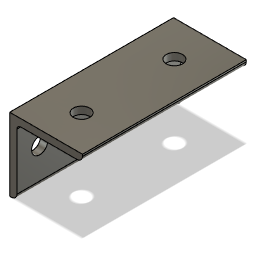
Equerre 80x80x8 longueur 180mm (Autodesk Fusion 360 design; units mm, degrees)
Autodesk Fusion 360 part; units mm, degrees
sketch "Sketch1" plane through (0, 0, 0) normal (0, 0, 1) x (1, 0, 0)
  line L0 (0, 0) -> (0, 80)
  line L1 (0, 80) -> (80, 80)
  line L2 (8, 6) -> (8, 68)
  line L3 (12, 72) -> (74, 72)
  line L4 (80, 78) -> (80, 80)
  line L5 (0, 0) -> (2, 0)
  arc A0 (74, 72) -> (80, 78) centre (74, 78) ccw
  arc A1 (2, 0) -> (8, 6) centre (2, 6) ccw
  arc A2 (12, 72) -> (8, 68) centre (12, 68) ccw
  dimension "d1" = 80
  dimension "d2" = 80
  dimension "d4" = 6
  dimension "d5" = 6
  dimension "d6" = 4
  constraint coincident L0.start L5.start
  constraint horizontal L1
  constraint vertical L0
  constraint perpendicular L1 L4
  constraint perpendicular L2 L5
  constraint parallel L0 L2
  constraint parallel L1 L3
  constraint tangent L3 A0
  constraint tangent L4 A0
  constraint tangent L2 A1
  constraint tangent L5 A1
  constraint tangent L2 A2
  constraint tangent L3 A2
  measures "d1" distance of L0.start L0.end
  measures "d2" distance of L0.end L1.end
  measures "d4" radius of A0
  measures "d5" radius of A1
  measures "d6" radius of A2
extrude "Extrude1" add sketch "Sketch1" along normal mid plane 180
sketch "Sketch2" plane through (0, 0, 0) normal (-1, 0, 0) x (0, 0, 1)
  line L0 (-90, 0) -> (90, 0) construction
  line L1 (90, 0) -> (90, 80) construction
  line L2 (90, 80) -> (-90, 80) construction
  line L3 (-90, 80) -> (-90, 0) construction
  line L4 (-90, 80) -> (90, 80) construction
  line L5 (-90, 0) -> (-90, 80) construction
  line L6 (-90, 0) -> (90, 0) construction
  line L7 (90, 80) -> (90, 0) construction
  line L8 (-90, 40) -> (90, 40) construction
  line L9 (0, 80) -> (0, 0) construction
  circle A0 centre (-65, 40) radius 9
  circle A1 centre (65, 40) radius 9
  dimension "d9" = 18
  dimension "d10" = 65
  constraint midpoint L3 L8.start
  constraint midpoint L1 L8.end
  constraint midpoint L4 L9.start
  constraint coincident L9.end origin
  constraint coincident L8 A0.centre
  constraint symmetric L9 A0 A1
  measures "d9" diameter of A0
  measures "d10" horizontal distance of L9.end A0.centre
extrude "Extrude2" cut sketch "Sketch2" against normal through all
sketch "Sketch3" plane through (0, 80, 0) normal (0, 1, 0) x (-1, 0, 0)
  line L0 (0, -90) -> (0, 90) construction
  line L1 (0, 90) -> (-80, 90) construction
  line L2 (-80, 90) -> (-80, -90) construction
  line L3 (-80, -90) -> (0, -90) construction
  line L4 (-80, 90) -> (0, 90) construction
  line L5 (-80, -90) -> (-80, 90) construction
  line L6 (0, -90) -> (0, 90) construction
  line L7 (0, -90) -> (-80, -90) construction
  line L8 (-80, 0) -> (0, 0) construction
  line L9 (-40, -90) -> (-40, 90) construction
  circle A0 centre (-40, -51) radius 9
  circle A1 centre (-40, 51) radius 9
  dimension "d12" = 18
  dimension "d13" = 51
  constraint midpoint L2 L8.start
  constraint coincident L8.end origin
  constraint midpoint L7 L9.start
  constraint midpoint L1 L9.end
  constraint coincident L9 A0.centre
  constraint symmetric L8 A0 A1
  measures "d12" diameter of A0
  measures "d13" distance of L8 A0.centre
extrude "Extrude3" cut sketch "Sketch3" against normal through all
equation "d13 = ( 102 / 2 ) * 1 mm"
